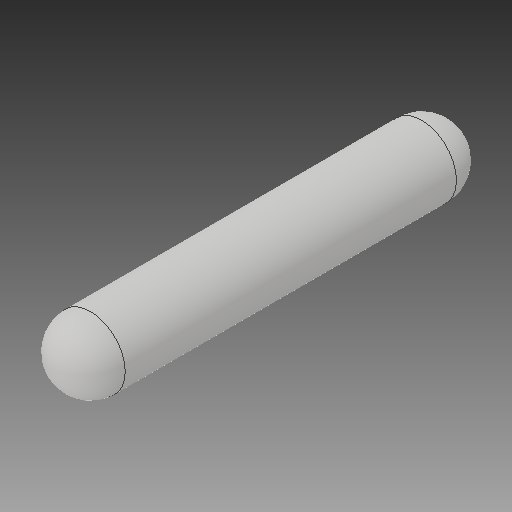
# Autodesk Inventor part: Pasador 2
Saved by Autodesk Inventor 2019 (Build 230136000, 136)
## iProperties
Created: 2019-07-01
Part Number: Pasador 2
Material: Generic
Document SubType Name: Modeling
Designer: Oscar Rojas
Density: 1 g/cm^3
Appearance: Default
Mass: 0.0340339 g
Surface Area: 0.722566 cm^2
Volume: 0.0340339 cm^3
Author: Oscar Rojas
Autodesk Inventor part; units mm, degrees
ref_plane "YZ Plane" through (0, 0, 0) normal (1, 0, 0) x (0, 1, 0)
ref_plane "XZ Plane" through (0, 0, 0) normal (0, 1, 0) x (-1, 0, 0)
ref_plane "XY Plane" through (0, 0, 0) normal (0, 0, 1) x (1, 0, 0)
sketch "Sketch1" plane through (0, 0, 0) normal (0, 0, 1) x (1, 0, 0)
  circle A0 centre (0, 0) radius 2
  dimension "d0" = 4
  constraints: 1 centre point, 1 coincident
  measures "d0" diameter of A0
extrude "Extrusion1" add sketch "Sketch1" along normal blind 23
fillet "Fillet1" radius 2 2 edges at (-2, 0, 23) (-2, 0, 0)
scale "Scale1" factors (0.5, 0.5, 0.5) then translate (0, 0, 5.75) bodies 1
body "Solid1"
